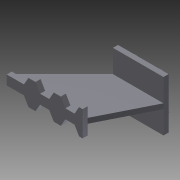
# Autodesk Inventor part: 3479
Saved by Autodesk Inventor 2011 SP1 (Build 150282100, 282)
## iProperties
Created: 2011-09-28
Part Number: 3479
Cost Center: 0 kg
Material: Steel
Document SubType Name: Modeling
Designer: PMe
Authority: 0 mm^3
Stock Number: =<Filenr>_<Document number>
Density: 7.85 g/cm^3
Company: Allseas Engineering BV
Subject: =<Title><TITLE 1_2> <TITLE 2_2>
Author: PMe
Act. Code: DW000
SaveDate: 2011-07-28
SaveTime: 18:32
FileName: Standard
TotalMass: 0 kg
TotalVolume: 0 mm^3
Autodesk Inventor part; units mm, degrees
ref_plane "YZ Plane" through (0, 0, 0) normal (1, 0, 0) x (0, 1, 0)
ref_plane "XZ Plane" through (0, 0, 0) normal (0, 1, 0) x (-1, 0, 0)
ref_plane "XY Plane" through (0, 0, 0) normal (0, 0, 1) x (1, 0, 0)
sketch "Sketch1" plane through (0, 0, 0) normal (0, 0, 1) x (1, 0, 0)
  line L0 (0, 0) -> (0, 1.6)
  line L1 (0, 1.6) -> (-24, 1.6)
  line L2 (-24, 1.6) -> (-24, 0)
  line L3 (-24, 0) -> (0, 0)
  line L4 (0, 1.6) -> (8, 17.6)
  line L5 (8, 17.6) -> (-8, 17.6)
  line L6 (-8, 17.6) -> (-24, 1.6)
  line L7 (-8, 17.6) -> (-8, 19.2)
  line L8 (-8, 19.2) -> (8, 19.2)
  line L9 (8, 19.2) -> (8, 17.6)
  dimension "d0" = 16
  dimension "d1" = 24
  dimension "d2" = 1.6
  dimension "d3" = 1.6
  dimension "d4" = 19.2
  dimension "d5" = 8
  constraints: 20 end point, 4 parallel, 3 perpendicular, 1 vertical
  measures "d0" distance of L7.end L8.end
  measures "d1" distance of L2.end L0.start
  measures "d2" distance of L1.end L2.end
  measures "d3" distance of L8.end L4.end
  measures "d4" distance between parallel lines of L8 L3
  measures "d5" distance between parallel lines of L9 L0
extrude "Extrusion1" add sketch "Sketch1" along normal mid plane 16 contours L5 L7 L8 L9
extrude "Extrusion2" add sketch "Sketch1" along normal mid plane 8 contours L3 L2 L1 L0
extrude "Extrusion3" add sketch "Sketch1" along normal mid plane 1.6 contours L1 L6 L5 L4
sketch "Sketch2" plane through (-8, 19.2, 8) normal (0, 1, 0) x (1, 0, 0)
  line L0 (16, 16) -> (0, 16) projected
  line L1 (0, 16) -> (0, 0) projected
  circle A0 centre (4, 12) radius 2.5
  circle A1 centre (4, 12) radius 1.5
  circle A2 centre (12, 12) radius 1.5
  circle A3 centre (12, 12) radius 2.5
  circle A4 centre (4, 4) radius 1.5
  circle A5 centre (4, 4) radius 2.5
  circle A6 centre (12, 4) radius 1.5
  circle A7 centre (12, 4) radius 2.5
  point P0 (8, 8)
  dimension "d12" = 5
  dimension "d13" = 4
  dimension "d14" = 8
  dimension "d15" = 4
  dimension "d16" = 8
  dimension "d17" = 3
  constraints: 8 centre point, 6 equal radius, 4 coincident, 2 horizontal alignment, 2 vertical alignment
  measures "d12" diameter of A5
  measures "d13" distance from line of L1 A0.centre
  measures "d14" distance of A2.centre A0.centre
  measures "d15" distance from line of L0 A0.centre
  measures "d16" distance of A4.centre A0.centre
  measures "d17" diameter of A4
extrude "Extrusion4" add sketch "Sketch2" along normal blind 1.6
sketch "Sketch3" plane through (-24, 0, 4) normal (0, -1, 0) x (1, 0, 0)
  line L0 (24, 0) -> (0, 0) projected
  line L1 (0, -8) -> (0, 0) projected
  line L2 (0, -8) -> (24, -8) projected
  line L3 (24, 0) -> (24, -8) projected
  line L4 (22.8868, 0) -> (21.4434, -2.5)
  line L5 (21.4434, -2.5) -> (18.5566, -2.5)
  line L6 (18.5566, -2.5) -> (17.1132, 0)
  circle A0 centre (20, 0) radius 2.5 construction
  line L7 (14.8868, 0) -> (13.4434, -2.5)
  line L8 (13.4434, -2.5) -> (10.5566, -2.5)
  line L9 (10.5566, -2.5) -> (9.1132, 0)
  circle A1 centre (12, 0) radius 2.5 construction
  line L10 (6.8868, 0) -> (5.4434, -2.5)
  line L11 (5.4434, -2.5) -> (2.5566, -2.5)
  line L12 (2.5566, -2.5) -> (1.1132, 0)
  circle A2 centre (4, 0) radius 2.5 construction
  line L13 (0, -4) -> (24, -4) construction
  line L14 (0, -4) -> (24, -4)
  line L15 (22.8868, -8) -> (21.4434, -5.5)
  line L16 (21.4434, -5.5) -> (18.5566, -5.5)
  line L17 (18.5566, -5.5) -> (17.1132, -8)
  line L18 (10.5566, -5.5) -> (9.1132, -8)
  line L19 (13.4434, -5.5) -> (10.5566, -5.5)
  line L20 (14.8868, -8) -> (13.4434, -5.5)
  line L21 (2.5566, -5.5) -> (1.1132, -8)
  line L22 (5.4434, -5.5) -> (2.5566, -5.5)
  line L23 (6.8868, -8) -> (5.4434, -5.5)
  line L24 (2.5566, -5.5) -> (0, -5.5)
  line L25 (2.5566, -2.5) -> (0, -2.5)
  line L26 (1.1132, -8) -> (6.8868, -8)
  line L27 (9.1132, -8) -> (14.8868, -8)
  line L28 (17.1132, -8) -> (22.8868, -8)
  line L29 (22.8868, 0) -> (17.1132, 0)
  line L30 (14.8868, 0) -> (9.1132, 0)
  line L31 (6.8868, 0) -> (1.1132, 0)
  line L32 (1.1132, 0) -> (0, 0)
  line L33 (0, 0) -> (0, -2.5)
  line L34 (0, -5.5) -> (0, -8)
  line L35 (0, -8) -> (1.1132, -8)
  point P0 (20, -8)
  point P1 (12, -8)
  point P2 (4, -8)
  dimension "d20" = 5
  dimension "d21" = 4
  dimension "d22" = 120
  dimension "d25" = 8
  constraints: 64 end point, 15 symmetric about line, 12 collinear, 6 point on line, 3 centre point, 3 tangent, 2 perpendicular, 1 equal length, 1 horizontal, 1 midpoint, 1 parallel, 18 other
  measures "d20" diameter of A0
  measures "d21" distance from line of L3 A0.centre
  measures "d22" angle of L0 L4
  measures "d25" distance of A0.centre A1.centre
extrude "Extrusion5" cut sketch "Sketch3" against normal blind 1.6 contours L4 L5 L6 L0 | L7 L8 L9 L0 | L2 L17 L16 L15 | L24 L21 L2 L1 | L1 L0 L12 L25 | L22 L23 L2 L21 | L12 L0 L10 L11 | L2 L18 L19 L20
body "Solid1"
